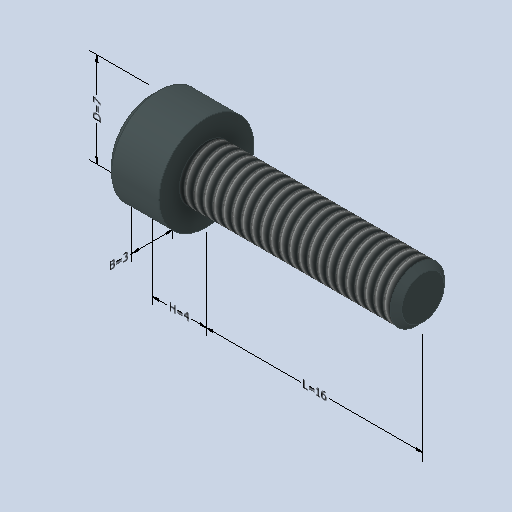
# Autodesk Inventor part: CBB4-16
Saved by Autodesk Inventor 2023 (Build 270158000, 158)
## iProperties
Category: PARTsolutions
Company: TOHATSU
Created: 2023-07-22
Part Number: CBB4-16
Material: Generic
Catalog Web Link: www.cadenas.de
Description: CBB-Hexagon socket screws
Vendor: TOHATSU
Document SubType Name: Modeling
Designer: psAdmin
Manufacturer: TOHATSU
Mass: 2.62195 g
Surface Area: 3.76612 cm^2
Volume: 0.335717 cm^3
Density: 7.81 g/cm^3
Appearance: PSOLRGB-76-89-91
PSOL_IDENT_0: {$CADENAS_DATA/23d-libs/tohatsu/spring_screw_washer/screws_bolts_nuts/screws_bolts/cbb.prj},153 {VTY
PSOL_IDENT_1: P=3D},{NB=CBB4-16},{LINA=CBB4-16},{NN=CBB},{DATE=19.07.2023 02:54:23},{GEOMDATE=08.12.2022 08:35:03}
PSOL_IDENT_2: ,{VERSION=},{LINEID=20},{WBVAR=L},{WBNUMERIC=L}  {NB=CBB4-16},{LINA=CBB4-16},{KT=DUMMY},{PN=CBB4-16}
PSOL_IDENT_3: ,{ROHS=YES},{TYPE=CBB},{MA=SCM435},{QU=7810},{M=4},{L=16},{DIML=5,6,8,10,12,16,20,25,30,35,40,45,50}
PSOL_IDENT_4: ,{P=0.70},{MXP=M4X0.7},{D=7.0},{H=4.0},{B=3.0},{C=16},{URL=https://www.tohatsu.com.tw},{WED=網站}
NB: CBB4-16
NN: CBB
NT: Hexagon socket screws
NBSYN: $PN.
LINA: CBB4-16
CATALOG: TOHATSU
PN: CBB4-16
ROHS: YES
MA: SCM435
M: 4
L: 16
WED: 網站
SUPPLIER: TOHATSU
ARTICLENO: CBB4-16
BOMINFO: CBB4-16
CREATOR: CADENAS GmbH
Title: CBB4-16
Author: Cadenas PARTsolutions
Comments: Hexagon socket screws
Autodesk Inventor part; units mm, degrees
sketch "__1" plane through (0, 0, 0) normal (0, 0, 1) x (1, 0, 0)
  line L0 (66, 0) -> (-66, 0)
  line L1 (0, 0) -> (0, 3.5)
  line L2 (0, 3.5) -> (4, 3.5)
  line L3 (4, 3.5) -> (4, 2)
  line L4 (4, 2) -> (19.5705, 2)
  line L5 (19.5705, 2) -> (20, 1.5705)
  line L6 (20, 1.5705) -> (20, 0)
  line L7 (20, 0) -> (0, 0)
  constraints: 16 end point
revolve "Revolution1" add sketch "__1" angle 360 about axis through (66, 0, 0) along (1, 0, 0)
thread "Thread1" size "M4x0.7" class "6g" standard "ISO Metric profile" full length
sketch "__2" plane through (0, 0, 0) normal (1, 0, 0) x (0, 0, -1)
  line L0 (-1.5, -0.866) -> (0, -1.7321)
  line L1 (0, -1.7321) -> (1.5, -0.866)
  line L2 (1.5, -0.866) -> (1.5, 0.866)
  line L3 (1.5, 0.866) -> (0, 1.7321)
  line L4 (0, 1.7321) -> (-1.5, 0.866)
  line L5 (-1.5, 0.866) -> (-1.5, -0.866)
  constraints: 12 end point
extrude "Extrusion1" cut sketch "__2" along normal blind 2
chamfer "Chamfer1" distance 0.5 angle 45 1 edges at (0, -3.5, 0)
ref_plane "PPBF_KEDS_XY" through (4, 0, 0) normal (-1, 0, 0) x (0, 0, -1)
ref_plane "PPBF_KEDS_YZ" through (4, 0, 0) normal (0, 0, -1) x (0, -1, 0)
ref_plane "PPBF_KEDS_ZX" through (4, 0, 0) normal (0, -1, 0) x (-1, 0, 0)
body "Solid1"
